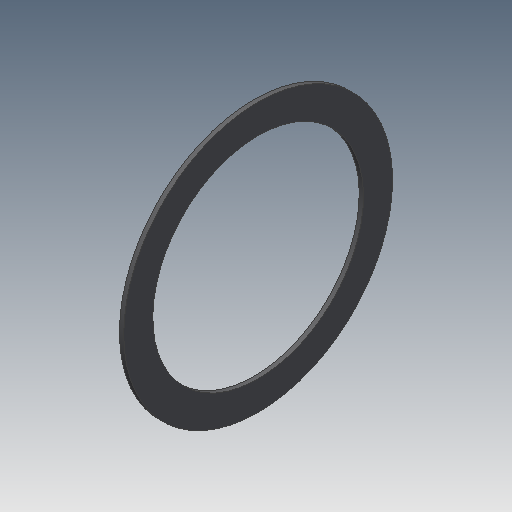
# Autodesk Inventor part: MF85ZZ Shield2
Saved by Autodesk Inventor 2019.4 (Build 234330000, 330)
## iProperties
Category: PARTsolutions
Company: NSK_RB
Created: 2019-11-12
Part Number: MF85ZZ Shield2
Material: 一般
Catalog Web Link: www.cadenas.de
Description: shielded_type_zz_zzs_S2-
Vendor: NSK_RB
Document SubType Name: Modeling
Designer: psadmin
Manufacturer: NSK_RB
Mass: 0.00194282 g
Surface Area: 0.380323 cm^2
Volume: 0.00194282 cm^3
Density: 1 g/cm^3
Appearance: PSOLRGB-128-128-128
PSOL_IDENT_0: {$CADENAS_DATA\23d-libs\nsk_rb\roller_bearings\deep_groove_bb\exstra_small_miniatur_bb\metric_design
PSOL_IDENT_1: _with_flange\shielded_type_zz_zzs_s2_1.prj},186 {VTYP=3D},{NB=MF85ZZ Shield2},{LINA=MF85ZZ Shield2},
PSOL_IDENT_2: {NN=shielded_type_zz_zzs_S2},{DATE=16.01.2019 01:41:17},{GEOMDATE=04.01.2008 00:00:00},{VERSION=},{L
PSOL_IDENT_3: INEID=210},{WBVAR=},{WBNUMERIC=}  {NB=MF85ZZ Shield2},{LINA=MF85ZZ Shield2},{KT=DUMMY},{IDNR=},{STAN=
PSOL_IDENT_4: },{ORDER=MF85ZZ},{SD=5.0},{X=5.0},{D=8},{DD=8},{DD1=0.0},{D2=9.2},{DD2=9.2},{B=0.0},{B1=2.5},{CC1=0.
PSOL_IDENT_5: 0},{C2=0.6},{CC2=0.6},{R=0.00},{R1=0.10},{DI1=5.80},{DI2=5.80},{SDE1=7.00},{SDE2=7.40},{CR1=310},{CO
PSOL_IDENT_6: R1=120},{CR2=31},{COR2=12.0},{LG=53000},{LO=63000},{DA=0.0},{DB=5.8},{RA=0.00},{RB=0.10},{MASS=0.41}
PSOL_IDENT_7: ,{SC=1}
NN: shielded_type_zz_zzs_S2
NB: MF85ZZ Shield2
NBSYN: $ORDER. Shield2
LINA: MF85ZZ Shield2
ORDER: MF85ZZ
SD: 5
X: 5
D: 8
DD: 8
DD1: 0
D2: 9.2
DD2: 9.2
B: 0
B1: 2.5
CC1: 0
C2: 0.6
CC2: 0.6
R: 0
R1: 0.1
DI1: 5.8
DI2: 5.8
SDE1: 7
SDE2: 7.4
CR1: 310
COR1: 120
CR2: 31
COR2: 12
LG: 53000
LO: 63000
DA: 0
DB: 5.8
RA: 0
RB: 0.1
MASS: 0.41
SC: 1
SUPPLIER: NSK_RB
ARTICLENO: MF85ZZ Shield2
BOMINFO: MF85ZZ Shield2
CREATOR: CADENAS GmbH
Title: MF85ZZ Shield2
Author: Cadenas PARTsolutions
Autodesk Inventor part; units mm, degrees
sketch "Sketch_1" plane through (0, 0, 0) normal (0, 0, 1) x (1, 0, 0)
  line L0 (2.4609, 0) -> (2.3438, 0)
  line L1 (2.3438, 2.9) -> (2.4609, 2.9)
  line L2 (2.4609, 2.9) -> (2.4609, 3.7)
  line L3 (2.4609, 3.7) -> (2.3438, 3.7)
  line L4 (2.3438, 3.7) -> (2.3438, 2.9)
  constraints: 10 end point
revolve "Revolution1" add sketch "Sketch_1" angle 360 about axis through (2.4609, 0, 0) along (1, 0, 0)
ref_plane "ip_st_1_XY" through (2.3438, 0, 0) normal (1, 0, 0) x (0, 0, -1)
ref_plane "ip_st_1_YZ" through (2.3438, 0, 0) normal (0, 0, -1) x (0, 1, 0)
ref_plane "ip_st_1_ZX" through (2.3438, 0, 0) normal (0, 1, 0) x (1, 0, 0)
body "Solid1"
